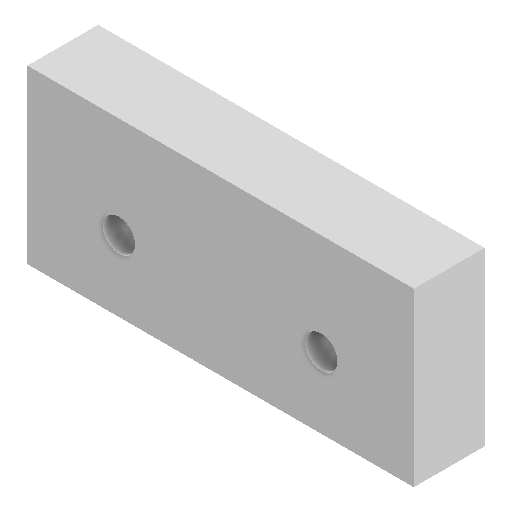
# Autodesk Inventor part: 00_Template_NEMA11_drill_holes_slider
Saved by Autodesk Inventor 2022 (Build 260153000, 153)
## iProperties
Created: 2023-06-26
Part Number: 00_Template_NEMA11_drill_holes_slider
Material: Generisch
Document SubType Name: Modeling
Designer: diederichbenedict
Density: 1 g/cm^3
Appearance: Vorgabe
Author: diederichbenedict
Autodesk Inventor part; units mm, degrees
ref_plane "YZ Plane" through (0, 0, 0) normal (1, 0, 0) x (0, 1, 0)
ref_plane "XZ Plane" through (0, 0, 0) normal (0, 1, 0) x (-1, 0, 0)
ref_plane "XY Plane" through (0, 0, 0) normal (0, 0, 1) x (1, 0, 0)
sketch "Skizze1" plane through (0, 0, 0) normal (0, 0, 1) x (1, 0, 0)
  line L0 (-3.3, -1) -> (-35.5, -1) projected
  line L1 (-35.5, 13) -> (-35.5, -1) projected
  line L2 (-3.3, 13) -> (-35.5, 13) projected
  line L3 (-3.3, 13) -> (-3.3, -1) projected
  circle A0 centre (-29.45, 6) radius 3.25 projected
  circle A1 centre (-9.45, 6) radius 3.25 projected
  line L4 (-38.5, 16) -> (-38.5, -4)
  line L5 (-38.5, -4) -> (-0.3, -4)
  line L6 (-0.3, -4) -> (-0.3, 16)
  line L7 (-0.3, 16) -> (-38.5, 16)
  circle A2 centre (-29.45, 6) radius 1.6
  circle A3 centre (-9.45, 6) radius 1.6
  line L8 (-38.5, -1) -> (-0.3, -1)
  point P0 (0, 0)
  dimension "d0" = 3
  dimension "d1" = 3.2
  dimension "d2" = 3.2
  constraints: 10 end point, 2 centre point, 2 coincident, 2 point on line, 1 horizontal, 3 other
  measures "d0" distance between parallel lines of L2 L7
  measures "d1" diameter of A2
  measures "d2" diameter of A3
extrude "Extrusion1" add sketch "Skizze1" along normal blind 3 contours L0 L1 L2 L3 | L3 L2 L1 L8 L4 L7 L6 | A0 | A1
sketch "Skizze2" plane through (0, 0, 0) normal (0, 0, -1) x (-1, 0, 0)
  line L0 (0.3, -1) -> (0.3, 16) projected
  line L1 (38.5, -1) -> (0.3, -1) projected
  line L2 (38.5, 16) -> (38.5, -1) projected
  line L3 (0.3, 16) -> (38.5, 16) projected
  circle A0 centre (9.45, 6) radius 1.6 projected
  circle A1 centre (29.45, 6) radius 1.6 projected
  line L4 (3.3, -1) -> (35.5, -1) construction
  line L5 (35.5, 13) -> (35.5, -1) construction
  line L6 (3.3, 13) -> (35.5, 13) construction
  line L7 (3.3, 13) -> (3.3, -1) construction
  line L8 (35.8, -1.3) -> (3, -1.3) construction
  line L9 (3, -1.3) -> (3, 13.3) construction
  line L10 (3, 13.3) -> (35.8, 13.3) construction
  line L11 (35.8, 13.3) -> (35.8, -1.3) construction
  line L12 (38.5, -1) -> (0.3, -1) projected
  line L13 (35.8, -1) -> (3, -1)
  line L14 (3, -1) -> (3, 13.3)
  line L15 (3, 13.3) -> (35.8, 13.3)
  line L16 (35.8, 13.3) -> (35.8, -1)
  point P0 (0, 0)
  point P1 (3, -1)
  dimension "d5" = 0.3
  constraints: 16 end point, 2 parallel, 2 point on line, 1 horizontal, 1 perpendicular, 3 other
  measures "d5" distance between parallel lines of L5 L11
extrude "Extrusion2" add sketch "Skizze2" along normal blind 4 contours L0 L3 L2 L1 L16 L15 L14
